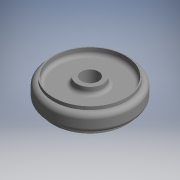
# Autodesk Inventor part: 2.00005.4411 1/4 (C)
Saved by Autodesk Inventor 2017.3 (Build 213256000, 256)
## iProperties
Part Number: 2.00005.4411 1/4 (C)
Material: Generic
Catalog Web Link: www.cadenas.de
Description: Performa Rubber C-Wheels - Capacity up to 1700 lbs Each
Vendor: COLSONGROUP
Document SubType Name: Modeling
Designer: partserver
Manufacturer: COLSONGROUP
Mass: 163.208 g
Surface Area: 364.55 cm^2
Volume: 163.208 cm^3
Density: 1 g/cm^3
Appearance: PSOLRGB-175-175-175
Category: PARTsolutions
Company: COLSONGROUP
Title: 2.00005.4411 1/4 (C)
Author: Cadenas PARTsolutions
Comments: Wheels - Capacity up to 1700 lbs Each
PSOL_IDENT_0: {$CADENAS_DATA\23d-libs\colsongroup\colson\wheels\performa_rubber\performa_rubber_core.prj},210 {VTY
PSOL_IDENT_1: P=3D},{NB=2.00005.4411 1/4 (C)},{LINA=2.00005.4411 1/4 (C)},{NN=Performa Rubber C},{DATE=10.12.2018
PSOL_IDENT_2: 11:02:41},{GEOMDATE=09.06.2017 06:04:28},{VERSION=},{LINEID=10},{WBVAR=WT,SER,D,W,WB,TG},{WBNUMERIC=
PSOL_IDENT_3: D,W}  {NB=2.00005.4411 1/4 (C)},{LINA=2.00005.4411 1/4 (C)},{KT=DUMMY},{PN=2.00005.4411 1/4},{WH=Per
PSOL_IDENT_4: forma Rubber},{WT=PRFG},{SER=2},{SERALG= '1','1 Series (Capacity up to 145 lbs)','2','2 Series (Capa
PSOL_IDENT_5: city up to 325 lbs)','3','3 Series (Capacity up to 375 lbs)','4','4 Series (Capacity up to 500 lbs)'
PSOL_IDENT_6: ,'5','5 Series (Capacity up to 675 lbs)' },{D=5},{DALG=2.5,3,3.5,4,5,6},{DPN=05},{W=1.25},{WALG=1.25
PSOL_IDENT_7: },{WTPN1=4},{WTPN2=4},{WTPN3=},{CAP=320},{CAPALG=320},{CAPPN=},{WB=1},{WBALG= '1','Delrin','5','Ball'
PSOL_IDENT_8: },{WBPN=441},{TG=},{TGALG= <'','None'>,' TG1','Metal (TG1)',' TG2','Plastic (TG2)' },{TGPN=},{BB=0.
PSOL_IDENT_9: 50000000},{LBB=0.90625000},{HUB=1.43750000},{SBB=0.37500000},{SBL=1.50000000},{WEIGHT=0.00000000},{C
PSOL_IDENT_10: ON=1},{D1=1.38},{D2=3.88},{BORE=0.895},{ANGS=6},{ANDT=3},{R1=0.25},{TT=0.28},{W1=0.175},{D3=3.7},{T=
PSOL_IDENT_11: 0.5},{ANGD=10},{ANGU=5},{T2=0.19},{T3=0.06},{CON2=4},{W2=1.25},{HUBR=1.25},{WR=0.9},{D4=4.44},{CPWB=
PSOL_IDENT_12: 0.625},{CPWB2=0.625},{TGCP=0.75},{SPCP=0.80375},{BORE2=1.5748},{BOREL=0.625}
NB: 2.00005.4411 1/4 (C)
NN: Performa Rubber C
NT: Wheels - Capacity up to 1700 lbs Each
NBSYN: $PN. (C)
LINA: 2.00005.4411 1/4 (C)
CATALOG: Colson Group
PN: 2.00005.4411 1/4
WH: Performa Rubber
WT: Flat Gray Thread
SER: 2 Series (Capacity up to 325 lbs)
D: 5
W: 0
CAP: 320
WB: Delrin
BB: 0
LBB: 0
HUB: 0
SBB: 0
SBL: 0
WEIGHT: 0
BORE: 0.895
SUPPLIER: COLSONGROUP
ARTICLENO: 2.00005.4411 1/4 (C)
BOMINFO: 2.00005.4411 1/4 (C)
CREATOR: CADENAS GmbH
Autodesk Inventor part; units mm, degrees
sketch "Sketch_20" plane through (0, 0, 0) normal (1, 0, 0) x (0, 1, 0)
  line L0 (0, -15.875) -> (0, 15.875)
  line L1 (0, 15.875) -> (17.526, 15.875)
  line L2 (17.526, 15.875) -> (17.526, 11.1125)
  arc A0 (17.526, 11.1125) -> (22.2885, 6.35) centre (22.2885, 11.1125) ccw
  line L3 (22.2885, 6.35) -> (42.9895, 6.35)
  arc A1 (42.9895, 6.35) -> (47.752, 11.1125) centre (42.9895, 11.1125) ccw
  line L4 (47.752, 11.1125) -> (47.752, 15.875)
  line L5 (47.752, 15.875) -> (49.276, 15.875)
  line L6 (49.276, 15.875) -> (49.276, 11.43)
  line L7 (49.276, 11.43) -> (50.038, 11.43)
  arc A2 (56.388, 5.08) -> (50.038, 11.43) centre (50.038, 5.08) ccw
  line L8 (56.388, 5.08) -> (56.388, -5.08)
  arc A3 (50.038, -11.43) -> (56.388, -5.08) centre (50.038, -5.08) ccw
  line L9 (50.038, -11.43) -> (49.276, -11.43)
  line L10 (49.276, -11.43) -> (49.276, -15.875)
  line L11 (49.276, -15.875) -> (47.752, -15.875)
  line L12 (47.752, -15.875) -> (47.752, -11.1125)
  arc A4 (47.752, -11.1125) -> (42.9895, -6.35) centre (42.9895, -11.1125) ccw
  line L13 (42.9895, -6.35) -> (22.2885, -6.35)
  arc A5 (22.2885, -6.35) -> (17.526, -11.1125) centre (22.2885, -11.1125) ccw
  line L14 (17.526, -11.1125) -> (17.526, -15.875)
  line L15 (17.526, -15.875) -> (0, -15.875)
  line L16 (0, -15.875) -> (0, 15.875)
  constraints: 34 end point, 12 point on circle, 6 centre point
revolve "Revolution1" add sketch "Sketch_20" angle 360 about axis through (0, 0, -15.875) along (0, 0, -1)
sketch "Sketch_3" plane through (0, 0, 0) normal (1, 0, 0) x (0, 1, 0)
  line L0 (0, -18.2563) -> (0, 18.2563)
  line L1 (0, 18.2563) -> (11.3665, 18.2563)
  line L2 (11.3665, 18.2563) -> (11.3665, -18.2563)
  line L3 (11.3665, -18.2563) -> (0, -18.2563)
  line L4 (0, -18.2563) -> (0, 18.2563)
  constraints: 10 end point
revolve "Revolution2" cut sketch "Sketch_3" angle 360 about axis through (0, 0, -18.2563) along (0, 0, -1)
ref_plane "BB_1_XY" through (0, 6.35, -18.2563) normal (1, 0, 0) x (0, 0, -1)
ref_plane "BB_1_YZ" through (0, 6.35, -18.2563) normal (0, 0, -1) x (0, 1, 0)
ref_plane "BB_1_ZX" through (0, 6.35, -18.2563) normal (0, 1, 0) x (1, 0, 0)
ref_plane "BB_2_XY" through (0, -6.35, -18.2563) normal (1, 0, 0) x (0, 0, -1)
ref_plane "BB_2_YZ" through (0, -6.35, -18.2563) normal (0, 0, -1) x (0, 1, 0)
ref_plane "BB_2_ZX" through (0, -6.35, -18.2563) normal (0, 1, 0) x (1, 0, 0)
ref_plane "D_1_XY" through (0, 63.5, 0) normal (0, 0, 1) x (1, 0, 0)
ref_plane "D_1_YZ" through (0, 63.5, 0) normal (1, 0, 0) x (0, 1, 0)
ref_plane "D_1_ZX" through (0, 63.5, 0) normal (0, 1, 0) x (0, 0, 1)
ref_plane "D_2_XY" through (0, -63.5, 0) normal (0, 0, 1) x (1, 0, 0)
ref_plane "D_2_YZ" through (0, -63.5, 0) normal (1, 0, 0) x (0, 1, 0)
ref_plane "D_2_ZX" through (0, -63.5, 0) normal (0, 1, 0) x (0, 0, 1)
ref_plane "HUB_1_XY" through (0, -17.526, 18.2563) normal (1, 0, 0) x (0, 0, -1)
ref_plane "HUB_1_YZ" through (0, -17.526, 18.2563) normal (0, 0, -1) x (0, 1, 0)
ref_plane "HUB_1_ZX" through (0, -17.526, 18.2563) normal (0, 1, 0) x (1, 0, 0)
ref_plane "HUB_2_XY" through (0, -17.526, -18.2563) normal (1, 0, 0) x (0, 0, -1)
ref_plane "HUB_2_YZ" through (0, -17.526, -18.2563) normal (0, 0, -1) x (0, 1, 0)
ref_plane "HUB_2_ZX" through (0, -17.526, -18.2563) normal (0, 1, 0) x (1, 0, 0)
ref_plane "W_1_XY" through (0, 17.526, 15.875) normal (1, 0, 0) x (0, 0, -1)
ref_plane "W_1_YZ" through (0, 17.526, 15.875) normal (0, 0, -1) x (0, 1, 0)
ref_plane "W_1_ZX" through (0, 17.526, 15.875) normal (0, 1, 0) x (1, 0, 0)
ref_plane "W_2_XY" through (0, 17.526, -15.875) normal (1, 0, 0) x (0, 0, -1)
ref_plane "W_2_YZ" through (0, 17.526, -15.875) normal (0, 0, -1) x (0, 1, 0)
ref_plane "W_2_ZX" through (0, 17.526, -15.875) normal (0, 1, 0) x (1, 0, 0)
ref_plane "core_XY" through (0, 0, 0) normal (0, 0, 1) x (1, 0, 0)
ref_plane "core_YZ" through (0, 0, 0) normal (1, 0, 0) x (0, 1, 0)
ref_plane "core_ZX" through (0, 0, 0) normal (0, 1, 0) x (0, 0, 1)
ref_plane "core_to_bearing1_XY" through (0, 0, 15.875) normal (0, 0, 1) x (1, 0, 0)
ref_plane "core_to_bearing1_YZ" through (0, 0, 15.875) normal (1, 0, 0) x (0, 1, 0)
ref_plane "core_to_bearing1_ZX" through (0, 0, 15.875) normal (0, 1, 0) x (0, 0, 1)
ref_plane "core_to_bearing2_XY" through (0, 0, -15.875) normal (0, 0, 1) x (1, 0, 0)
ref_plane "core_to_bearing2_YZ" through (0, 0, -15.875) normal (1, 0, 0) x (0, 1, 0)
ref_plane "core_to_bearing2_ZX" through (0, 0, -15.875) normal (0, 1, 0) x (0, 0, 1)
ref_plane "core_to_tg1_XY" through (0, 0, 19.05) normal (0, 0, 1) x (1, 0, 0)
ref_plane "core_to_tg1_YZ" through (0, 0, 19.05) normal (1, 0, 0) x (0, 1, 0)
ref_plane "core_to_tg1_ZX" through (0, 0, 19.05) normal (0, 1, 0) x (0, 0, 1)
ref_plane "core_to_tg2_XY" through (0, 0, -19.05) normal (0, 0, 1) x (1, 0, 0)
ref_plane "core_to_tg2_YZ" through (0, 0, -19.05) normal (1, 0, 0) x (0, 1, 0)
ref_plane "core_to_tg2_ZX" through (0, 0, -19.05) normal (0, 1, 0) x (0, 0, 1)
ref_plane "to_spacer1_XY" through (0, 0, 20.4153) normal (0, 0, 1) x (1, 0, 0)
ref_plane "to_spacer1_YZ" through (0, 0, 20.4153) normal (1, 0, 0) x (0, 1, 0)
ref_plane "to_spacer1_ZX" through (0, 0, 20.4153) normal (0, 1, 0) x (0, 0, 1)
ref_plane "to_spacer2_XY" through (0, 0, -20.4153) normal (0, 0, 1) x (1, 0, 0)
ref_plane "to_spacer2_YZ" through (0, 0, -20.4153) normal (1, 0, 0) x (0, 1, 0)
ref_plane "to_spacer2_ZX" through (0, 0, -20.4153) normal (0, 1, 0) x (0, 0, 1)
ref_plane "to_washer1_XY" through (0, 0, 18.2563) normal (0, 0, 1) x (1, 0, 0)
ref_plane "to_washer1_YZ" through (0, 0, 18.2563) normal (1, 0, 0) x (0, 1, 0)
ref_plane "to_washer1_ZX" through (0, 0, 18.2563) normal (0, 1, 0) x (0, 0, 1)
ref_plane "to_washer2_XY" through (0, 0, -18.2563) normal (0, 0, 1) x (1, 0, 0)
ref_plane "to_washer2_YZ" through (0, 0, -18.2563) normal (1, 0, 0) x (0, 1, 0)
ref_plane "to_washer2_ZX" through (0, 0, -18.2563) normal (0, 1, 0) x (0, 0, 1)
body "Solid1"
